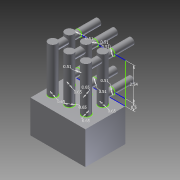
# Autodesk Inventor part: pin_socket
Saved by Autodesk Inventor 2012 (Build 160160000, 160)
## iProperties
Created: 2014-09-03
Part Number: pin_socket
Material: Default
Document SubType Name: Modeling
Designer: hannes.maierflaig
Density: 1 g/cm^3
Author: hannes.maierflaig
Autodesk Inventor part; units mm, degrees
ref_plane "YZ Plane" through (0, 0, 0) normal (1, 0, 0) x (0, 1, 0)
ref_plane "XZ Plane" through (0, 0, 0) normal (0, 1, 0) x (-1, 0, 0)
ref_plane "XY Plane" through (0, 0, 0) normal (0, 0, 1) x (1, 0, 0)
sketch "Skizze1" plane through (0, 0, 0) normal (0, 0, 1) x (1, 0, 0)
  line L0 (0, 0) -> (4.19, 0)
  line L1 (4.19, 0) -> (4.19, 3.05)
  line L2 (4.19, 3.05) -> (0, 3.05)
  line L3 (0, 3.05) -> (0, 0)
  dimension "d0" = 4.19
  dimension "d1" = 3.05
  constraints: 8 end point, 2 parallel, 1 horizontal, 1 perpendicular
  measures "d0" distance of L2.end L1.end
  measures "d1" distance of L1.end L0.end
extrude "Extrusion1" add sketch "Skizze1" along normal blind 2.5
sketch "Skizze2" plane through (0, 0, 2.5) normal (0, 0, 1) x (1, 0, 0)
  circle A0 centre (0.635, 2.335) radius 0.325
  circle A1 centre (0.635, 1.065) radius 0.325
  circle A2 centre (1.905, 2.335) radius 0.325
  circle A3 centre (1.905, 1.065) radius 0.325
  circle A4 centre (3.175, 1.065) radius 0.325
  circle A5 centre (3.175, 2.335) radius 0.325
  dimension "d4" = 0.65
  dimension "d5" = 0.65
  dimension "d6" = 0.65
  dimension "d7" = 0.65
  dimension "d8" = 0.65
  dimension "d9" = 0.65
  constraints: 9 coincident, 6 centre point
  measures "d4" diameter of A0
  measures "d5" diameter of A1
  measures "d6" diameter of A2
  measures "d7" diameter of A3
  measures "d8" diameter of A4
  measures "d9" diameter of A5
extrude "Extrusion2" add sketch "Skizze2" along normal blind 2.35 and the other way blind 6 separate body
combine bodies "Kombinieren2" operation type subtract main body 1 bodies to subtract 2
extrude "Extrusion4" add sketch "Skizze2" along normal blind 3.5 bodies 1
sketch "Skizze4" plane through (0, 3.05, 0) normal (0, 1, 0) x (1, 0, 0)
  line L0 (0, -2.5) -> (4.19, -2.5)
  line L1 (4.19, -2.5) -> (4.19, -3)
  line L2 (4.19, -3) -> (0, -3)
  line L3 (0, -3) -> (0, -2.5)
  line L4 (0, -3) -> (4.19, -3)
  line L5 (4.19, -3) -> (4.19, -5.54)
  line L6 (4.19, -5.54) -> (0, -5.54)
  line L7 (0, -5.54) -> (0, -3)
  circle A0 centre (0.6, -5.54) radius 0.255
  circle A1 centre (1.87, -5.54) radius 0.255
  circle A2 centre (3.14, -5.54) radius 0.255
  circle A3 centre (3.14, -3) radius 0.255
  circle A4 centre (1.87, -3) radius 0.255
  circle A5 centre (0.6, -3) radius 0.255
  point P0 (0.6, -0.46)
  dimension "d18" = 0.5
  dimension "d19" = 2.54
  dimension "d20" = 0.51
  dimension "d21" = 0.51
  dimension "d22" = 0.51
  dimension "d23" = 0.51
  dimension "d24" = 0.51
  dimension "d25" = 0.51
  constraints: 16 end point, 6 centre point, 6 coincident, 5 point on line, 4 parallel, 2 horizontal, 2 perpendicular
  measures "d18" distance of L0.end L1.end
  measures "d19" distance of L4.end L5.end
  measures "d20" diameter of A0
  measures "d21" diameter of A1
  measures "d22" diameter of A2
  measures "d23" diameter of A3
  measures "d24" diameter of A4
  measures "d25" diameter of A5
extrude "Extrusion5" add sketch "Skizze4" against normal blind 2 and the other way blind 1.5 contours A0 L6 | L6 A0 | A2 L6 | L6 A2 | A1 L6 | L6 A1 bodies 1
extrude "Extrusion6" add sketch "Skizze4" against normal blind 0.75 and the other way blind 1.5 contours A5 L2 | L2 A5 | A3 L2 | L2 A3 | A4 L2 | L2 A4 bodies 1
